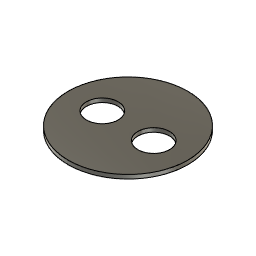
base_plate (Autodesk Fusion 360 design; units mm, degrees)
Autodesk Fusion 360 part; units mm, degrees
sketch "Sketch1" plane through (0, 0, 0) normal (0, 0, 1) x (1, 0, 0)
  circle A0 centre (0, 0) radius 30.2
  line L0 (0, 0) -> (13, 0) construction
  circle A1 centre (13, 0) radius 8
  line L1 (0, 0) -> (0, 6.6641) construction
  circle A2 centre (-13, 0) radius 8
  dimension "d1" = 60.4
  dimension "d2" = 13
  dimension "d3" = 16
  constraint coincident A0.centre L0.start
  constraint horizontal L0
  constraint coincident L0.end A1.centre
  constraint perpendicular L0 L1
  constraint symmetric A1 L1 A2
  measures "d1" diameter of A0
  measures "d2" distance of A0.centre L0.end
  measures "d3" diameter of A1
extrude "Extrude1" add sketch "Sketch1" along normal blind 2
equation "d2 = 5 mm + 8 mm"
